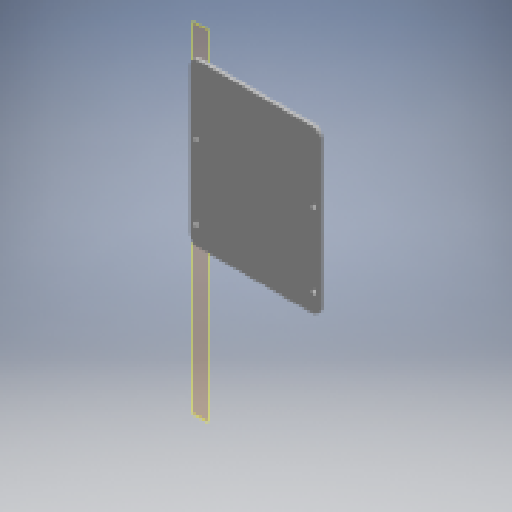
# Autodesk Inventor part: Poly3
Saved by Autodesk Inventor 2026.1 (Build 301233000, 233)
## iProperties
Created: 2025-09-25
Part Number: Poly3
Material: Polycarbonate, Smoke
Document SubType Name: Modeling
Designer: Teddy
Density: 1.2 g/cm^3
Appearance: Polycarbonate - Smoked
Author: Teddy
Autodesk Inventor part; units mm, degrees
ref_plane "YZ Plane" through (0, 0, 0) normal (1, 0, 0) x (0, 1, 0)
ref_plane "XZ Plane" through (0, 0, 0) normal (0, 1, 0) x (-1, 0, 0)
ref_plane "XY Plane" through (0, 0, 0) normal (0, 0, 1) x (1, 0, 0)
ref_plane "Work Plane1" through (0, 0, 0) normal (0, 0, 1) x (1, 0, 0)
sketch "Sketch1" plane through (0, 0, 0) normal (0, 0, 1) x (1, 0, 0)
  line L0 (-4.3544, 38.3987) -> (107.4056, 38.3987)
  line L1 (107.4056, 38.3987) -> (107.4056, 133.6487)
  line L2 (107.4056, 133.6487) -> (-4.3544, 133.6487)
  line L3 (-4.3544, 133.6487) -> (-4.3544, 38.3987)
  circle A0 centre (0.7751, 50.8) radius 2.1844
  circle A1 centre (102.3751, 50.8) radius 2.1844
  circle A2 centre (0.7751, 114.3) radius 2.1844
  circle A3 centre (102.3751, 114.3) radius 2.1844
  point P0 (0, 0)
  dimension "d0" = 111.76
  dimension "d1" = 95.25
  constraints: 8 end point, 4 centre point, 2 parallel, 1 horizontal, 1 perpendicular
  measures "d0" distance of L0.start L0.end
  measures "d1" distance of L2.end L0.start
extrude "Extrusion1" add sketch "Sketch1" along normal blind 3.175
fillet "Fillet1" radius 6.35 4 edges at (-4.3544, 38.3987, 1.5875) (107.4056, 38.3987, 1.5875) (-4.3544, 133.6487, 1.5875) (107.4056, 133.6487, 1.5875)
body "Solid1"
